Autodesk Fusion 360 part; units mm, degrees
(part 6 of 8)
  line L844 (-117.8501, 180.3501, -3) -> (-114.8501, 180.3501, -3)
  line L845 (-114.8501, 180.3501, -3) -> (-114.8501, 177.3501, -3)
  line L846 (-114.8501, 177.3501, -3) -> (-111.8501, 177.3501, -3)
  line L847 (-111.8501, 177.3501, -3) -> (-111.8501, 180.3501, -3)
  line L848 (-111.8501, 180.3501, -3) -> (-108.8501, 180.3501, -3)
  line L849 (-108.8501, 180.3501, -3) -> (-108.8501, 177.3501, -3)
  line L850 (-108.8501, 177.3501, -3) -> (-105.8501, 177.3501, -3)
  line L851 (-105.8501, 177.3501, -3) -> (-105.8501, 180.3501, -3)
  line L852 (-105.8501, 180.3501, -3) -> (-102.8501, 180.3501, -3)
  line L853 (-102.8501, 180.3501, -3) -> (-102.8501, 177.3501, -3)
  line L854 (-102.8501, 177.3501, -3) -> (-99.8501, 177.3501, -3)
  line L855 (-99.8501, 177.3501, -3) -> (-99.8501, 180.3501, -3)
  line L856 (-99.8501, 180.3501, -3) -> (-96.8501, 180.3501, -3)
  line L857 (-96.8501, 180.3501, -3) -> (-96.8501, 177.3501, -3)
  line L858 (-96.8501, 177.3501, -3) -> (-93.8501, 177.3501, -3)
  line L859 (-93.8501, 177.3501, -3) -> (-93.8501, 180.3501, -3)
  line L860 (-93.8501, 180.3501, -3) -> (-90.8501, 180.3501, -3)
  line L861 (-90.8501, 180.3501, -3) -> (-90.8501, 177.3501, -3)
  line L862 (-90.8501, 177.3501, -3) -> (-87.8501, 177.3501, -3)
  line L863 (-87.8501, 177.3501, -3) -> (-87.8501, 180.3501, -3)
  line L864 (-87.8501, 180.3501, -3) -> (-84.8501, 180.3501, -3)
  line L865 (-84.8501, 180.3501, -3) -> (-84.8501, 177.3501, -3)
  line L866 (-84.8501, 177.3501, -3) -> (-81.8501, 177.3501, -3)
  line L867 (-81.8501, 177.3501, -3) -> (-81.8501, 180.3501, -3)
  line L868 (-81.8501, 180.3501, -3) -> (-78.8501, 180.3501, -3)
  line L869 (-78.8501, 180.3501, -3) -> (-78.8501, 177.3501, -3)
  line L870 (-78.8501, 177.3501, -3) -> (-75.8501, 177.3501, -3)
  line L871 (-75.8501, 177.3501, -3) -> (-75.8501, 180.3501, -3)
  line L872 (-75.8501, 180.3501, -3) -> (-72.8501, 180.3501, -3)
  line L873 (-72.8501, 180.3501, -3) -> (-72.8501, 177.3501, -3)
  line L874 (-72.8501, 177.3501, -3) -> (-69.8501, 177.3501, -3)
  line L875 (-69.8501, 177.3501, -3) -> (-69.8501, 180.3501, -3)
  line L876 (-69.8501, 180.3501, -3) -> (-66.8501, 180.3501, -3)
  line L877 (-66.8501, 180.3501, -3) -> (-66.8501, 177.3501, -3)
  line L878 (-66.8501, 177.3501, -3) -> (-63.8501, 177.3501, -3)
  line L879 (-63.8501, 177.3501, -3) -> (-63.8501, 180.3501, -3)
  line L880 (-63.8501, 180.3501, -3) -> (-60.8501, 180.3501, -3)
  line L881 (-60.8501, 180.3501, -3) -> (-60.8501, 177.3501, -3)
  line L882 (-60.8501, 177.3501, -3) -> (-57.85, 177.3501, -3)
  line L883 (-57.85, 177.3501, -3) -> (-57.85, 180.3501, -3)
  line L884 (-57.85, 180.3501, -3) -> (-54.85, 180.3501, -3)
  line L885 (-54.85, 180.3501, -3) -> (-54.85, 177.3501, -3)
  line L886 (-54.85, 177.3501, -3) -> (-51.85, 177.3501, -3)
  line L887 (-51.85, 177.3501, -3) -> (-51.85, 180.3501, -3)
  line L888 (-51.85, 180.3501, -3) -> (-48.85, 180.3501, -3)
  line L889 (-48.85, 180.3501, -3) -> (-48.85, 177.3501, -3)
  line L890 (-48.85, 177.3501, -3) -> (-45.85, 177.3501, -3)
  line L891 (-45.85, 177.3501, -3) -> (-45.85, 180.3501, -3)
  line L892 (-45.85, 180.3501, -3) -> (-42.85, 180.3501, -3)
  line L893 (-42.85, 180.3501, -3) -> (-42.85, 177.3501, -3)
  line L894 (-42.85, 177.3501, -3) -> (-39.85, 177.3501, -3)
  line L895 (-39.85, 177.3501, -3) -> (-39.85, 180.3501, -3)
  line L896 (-39.85, 180.3501, -3) -> (-36.85, 180.3501, -3)
  line L897 (-36.85, 180.3501, -3) -> (-36.85, 177.3501, -3)
  line L898 (-36.85, 177.3501, -3) -> (-33.85, 177.3501, -3)
  line L899 (-33.85, 177.3501, -3) -> (-33.85, 180.3501, -3)
  line L900 (-33.85, 180.3501, -3) -> (-30.85, 180.3501, -3)
  line L901 (-30.85, 180.3501, -3) -> (-30.85, 177.3501, -3)
  line L902 (-30.85, 177.3501, -3) -> (-27.85, 177.3501, -3)
  line L903 (-27.85, 177.3501, -3) -> (-27.85, 180.3501, -3)
  line L904 (-27.85, 180.3501, -3) -> (-24.85, 180.3501, -3)
  line L905 (-24.85, 180.3501, -3) -> (-24.85, 177.3501, -3)
  line L906 (-24.85, 177.3501, -3) -> (-21.85, 177.3501, -3)
  line L907 (-21.85, 177.3501, -3) -> (-21.85, 180.3501, -3)
  line L908 (-21.85, 180.3501, -3) -> (-18.85, 180.3501, -3)
  line L909 (-18.85, 180.3501, -3) -> (-18.85, 177.3501, -3)
  line L910 (-18.85, 177.3501, -3) -> (-15.85, 177.3501, -3)
  line L911 (-15.85, 177.3501, -3) -> (-15.85, 180.3501, -3)
  line L912 (-15.85, 180.3501, -3) -> (-11.1, 180.3501, -3)
  line L913 (-11.1, 180.3501, -3) -> (-11.1, 177.3501, -3)
  line L914 (-11.1, 177.3501, -3) -> (-9.35, 177.3501, -3)
  line L915 (-9.35, 177.3501, -3) -> (-9.35, 176.6001, -3)
  line L916 (-9.35, 176.6001, -3) -> (-6.35, 176.6001, -3)
  line L917 (-6.35, 176.6001, -3) -> (-6.35, 172.8501, -3)
  line L918 (-6.35, 172.8501, -3) -> (-9.35, 172.8501, -3)
  line L919 (-9.35, 172.8501, -3) -> (-9.35, 169.8501, -3)
  line L920 (-9.35, 169.8501, -3) -> (-6.35, 169.8501, -3)
  line L921 (-6.35, 169.8501, -3) -> (-6.35, 166.8501, -3)
  line L922 (-6.35, 166.8501, -3) -> (-9.35, 166.8501, -3)
  line L923 (-9.35, 166.8501, -3) -> (-9.35, 163.8501, -3)
  line L924 (-9.35, 163.8501, -3) -> (-6.35, 163.8501, -3)
  line L925 (-6.35, 163.8501, -3) -> (-6.35, 160.8501, -3)
  line L926 (-6.35, 160.8501, -3) -> (-9.35, 160.8501, -3)
  line L927 (-9.35, 160.8501, -3) -> (-9.35, 157.8501, -3)
  line L928 (-9.35, 157.8501, -3) -> (-6.35, 157.8501, -3)
  line L929 (-6.35, 157.8501, -3) -> (-6.35, 154.8501, -3)
  line L930 (-6.35, 154.8501, -3) -> (-9.35, 154.8501, -3)
  line L931 (-9.35, 154.8501, -3) -> (-9.35, 151.8501, -3)
  line L932 (-9.35, 151.8501, -3) -> (-6.35, 151.8501, -3)
  line L933 (-6.35, 151.8501, -3) -> (-6.35, 148.8501, -3)
  line L934 (-6.35, 148.8501, -3) -> (-9.35, 148.8501, -3)
  line L935 (-9.35, 148.8501, -3) -> (-9.35, 145.8501, -3)
  line L936 (-9.35, 145.8501, -3) -> (-6.35, 145.8501, -3)
  line L937 (-6.35, 145.8501, -3) -> (-6.35, 142.8501, -3)
  line L938 (-6.35, 142.8501, -3) -> (-9.35, 142.8501, -3)
  line L939 (-9.35, 142.8501, -3) -> (-9.35, 139.8501, -3)
  line L940 (-9.35, 139.8501, -3) -> (-6.35, 139.8501, -3)
  line L941 (-6.35, 139.8501, -3) -> (-6.35, 136.8501, -3)
  line L942 (-6.35, 136.8501, -3) -> (-9.35, 136.8501, -3)
  line L943 (-9.35, 136.8501, -3) -> (-9.35, 133.8501, -3)
  line L944 (-9.35, 133.8501, -3) -> (-6.35, 133.8501, -3)
  line L945 (-6.35, 133.8501, -3) -> (-6.35, 130.8501, -3)
  line L946 (-6.35, 130.8501, -3) -> (-9.35, 130.8501, -3)
  line L947 (-9.35, 130.8501, -3) -> (-9.35, 127.8501, -3)
  line L948 (-9.35, 127.8501, -3) -> (-6.35, 127.8501, -3)
  line L949 (-6.35, 127.8501, -3) -> (-6.35, 124.8501, -3)
  line L950 (-6.35, 124.8501, -3) -> (-9.35, 124.8501, -3)
  line L951 (-9.35, 124.8501, -3) -> (-9.35, 121.8501, -3)
  line L952 (-9.35, 121.8501, -3) -> (-6.35, 121.8501, -3)
  line L953 (-6.35, 121.8501, -3) -> (-6.35, 118.8501, -3)
  line L954 (-6.35, 118.8501, -3) -> (-9.35, 118.8501, -3)
  line L955 (-9.35, 118.8501, -3) -> (-9.35, 115.8501, -3)
  line L956 (-9.35, 115.8501, -3) -> (-6.35, 115.8501, -3)
  line L957 (-6.35, 115.8501, -3) -> (-6.35, 112.8501, -3)
  line L958 (-6.35, 112.8501, -3) -> (-9.35, 112.8501, -3)
  line L959 (-9.35, 112.8501, -3) -> (-9.35, 109.8501, -3)
  line L960 (-9.35, 109.8501, -3) -> (-6.35, 109.8501, -3)
  line L961 (-6.35, 109.8501, -3) -> (-6.35, 106.8501, -3)
  line L962 (-6.35, 106.8501, -3) -> (-9.35, 106.8501, -3)
  line L963 (-9.35, 106.8501, -3) -> (-9.35, 103.8501, -3)
  line L964 (-9.35, 103.8501, -3) -> (-6.35, 103.8501, -3)
  line L965 (-6.35, 103.8501, -3) -> (-6.35, 100.8501, -3)
  line L966 (-6.35, 100.8501, -3) -> (-9.35, 100.8501, -3)
  line L967 (-9.35, 100.8501, -3) -> (-9.35, 97.8501, -3)
  line L968 (-9.35, 97.8501, -3) -> (-6.35, 97.8501, -3)
  line L969 (-6.35, 97.8501, -3) -> (-6.35, 94.8501, -3)
  line L970 (-6.35, 94.8501, -3) -> (-9.35, 94.8501, -3)
  line L971 (-9.35, 94.8501, -3) -> (-9.35, 91.8501, -3)
  line L972 (-9.35, 91.8501, -3) -> (-6.35, 91.8501, -3)
  line L973 (-6.35, 91.8501, -3) -> (-6.35, 88.8501, -3)
  line L974 (-6.35, 88.8501, -3) -> (-9.35, 88.8501, -3)
  line L975 (-9.35, 88.8501, -3) -> (-9.35, 85.8501, -3)
  line L976 (-9.35, 85.8501, -3) -> (-6.35, 85.8501, -3)
  line L977 (-6.35, 85.8501, -3) -> (-6.35, 82.8501, -3)
  line L978 (-6.35, 82.8501, -3) -> (-9.35, 82.8501, -3)
  line L979 (-9.35, 82.8501, -3) -> (-9.35, 79.8501, -3)
  line L980 (-9.35, 79.8501, -3) -> (-6.35, 79.8501, -3)
  line L981 (-6.35, 79.8501, -3) -> (-6.35, 76.8501, -3)
  line L982 (-6.35, 76.8501, -3) -> (-9.35, 76.8501, -3)
  line L983 (-9.35, 76.8501, -3) -> (-9.35, 73.8501, -3)
  line L984 (-9.35, 73.8501, -3) -> (-6.35, 73.8501, -3)
  line L985 (-6.35, 73.8501, -3) -> (-6.35, 70.8501, -3)
  line L986 (-6.35, 70.8501, -3) -> (-9.35, 70.8501, -3)
  line L987 (-9.35, 70.8501, -3) -> (-9.35, 67.8501, -3)
  line L988 (-9.35, 67.8501, -3) -> (-6.35, 67.8501, -3)
  line L989 (-6.35, 67.8501, -3) -> (-6.35, 64.8501, -3)
  line L990 (-6.35, 64.8501, -3) -> (-9.35, 64.8501, -3)
  line L991 (-9.35, 64.8501, -3) -> (-9.35, 61.8501, -3)
  line L992 (-9.35, 61.8501, -3) -> (-6.35, 61.8501, -3)
  line L993 (-6.35, 61.8501, -3) -> (-6.35, 58.85, -3)
  line L994 (-6.35, 58.85, -3) -> (-9.35, 58.85, -3)
  line L995 (-9.35, 58.85, -3) -> (-9.35, 55.85, -3)
  line L996 (-9.35, 55.85, -3) -> (-6.35, 55.85, -3)
  line L997 (-6.35, 55.85, -3) -> (-6.35, 52.85, -3)
  line L998 (-6.35, 52.85, -3) -> (-9.35, 52.85, -3)
  line L999 (-9.35, 52.85, -3) -> (-9.35, 49.85, -3)
  line L1000 (-9.35, 49.85, -3) -> (-6.35, 49.85, -3)
  line L1001 (-6.35, 49.85, -3) -> (-6.35, 46.85, -3)
  line L1002 (-6.35, 46.85, -3) -> (-9.35, 46.85, -3)
  line L1003 (-9.35, 46.85, -3) -> (-9.35, 43.85, -3)
  line L1004 (-9.35, 43.85, -3) -> (-6.35, 43.85, -3)
  line L1005 (-6.35, 43.85, -3) -> (-6.35, 40.85, -3)
  line L1006 (-6.35, 40.85, -3) -> (-9.35, 40.85, -3)
  line L1007 (-9.35, 40.85, -3) -> (-9.35, 37.85, -3)
  line L1008 (-9.35, 37.85, -3) -> (-6.35, 37.85, -3)
  line L1009 (-6.35, 37.85, -3) -> (-6.35, 34.85, -3)
  line L1010 (-6.35, 34.85, -3) -> (-9.35, 34.85, -3)
  line L1011 (-9.35, 34.85, -3) -> (-9.35, 31.85, -3)
  line L1012 (-9.35, 31.85, -3) -> (-6.35, 31.85, -3)
  line L1013 (-6.35, 31.85, -3) -> (-6.35, 28.1, -3)
  line L1014 (-6.35, 28.1, -3) -> (-9.35, 28.1, -3)
  line L1015 (-9.35, 28.1, -3) -> (-9.35, 27.35, -3)
  line L1016 (-9.35, 27.35, -3) -> (-11.1, 27.35, -3)
  line L1017 (-11.1, 27.35, -3) -> (-11.1, 24.35, -3)
  line L1018 (-11.1, 24.35, -3) -> (-15.85, 24.35, -3)
  line L1019 (-15.85, 24.35, -3) -> (-15.85, 27.35, -3)
  line L1020 (-15.85, 27.35, -3) -> (-18.85, 27.35, -3)
  line L1021 (-18.85, 27.35, -3) -> (-18.85, 24.35, -3)
  line L1022 (-18.85, 24.35, -3) -> (-21.85, 24.35, -3)
  line L1023 (-21.85, 24.35, -3) -> (-21.85, 27.35, -3)
  line L1024 (-21.85, 27.35, -3) -> (-24.85, 27.35, -3)
  line L1025 (-24.85, 27.35, -3) -> (-24.85, 24.35, -3)
  line L1026 (-24.85, 24.35, -3) -> (-27.85, 24.35, -3)
  line L1027 (-27.85, 24.35, -3) -> (-27.85, 27.35, -3)
  line L1028 (-27.85, 27.35, -3) -> (-30.85, 27.35, -3)
  line L1029 (-30.85, 27.35, -3) -> (-30.85, 24.35, -3)
  line L1030 (-30.85, 24.35, -3) -> (-33.85, 24.35, -3)
  line L1031 (-33.85, 24.35, -3) -> (-33.85, 27.35, -3)
  line L1032 (-33.85, 27.35, -3) -> (-36.85, 27.35, -3)
  line L1033 (-36.85, 27.35, -3) -> (-36.85, 24.35, -3)
  line L1034 (-36.85, 24.35, -3) -> (-39.85, 24.35, -3)
  line L1035 (-39.85, 24.35, -3) -> (-39.85, 27.35, -3)
  line L1036 (-39.85, 27.35, -3) -> (-42.85, 27.35, -3)
  line L1037 (-42.85, 27.35, -3) -> (-42.85, 24.35, -3)
  line L1038 (-42.85, 24.35, -3) -> (-45.85, 24.35, -3)
  line L1039 (-45.85, 24.35, -3) -> (-45.85, 27.35, -3)
  line L1040 (-45.85, 27.35, -3) -> (-48.85, 27.35, -3)
  line L1041 (-48.85, 27.35, -3) -> (-48.85, 24.35, -3)
  line L1042 (-48.85, 24.35, -3) -> (-51.85, 24.35, -3)
  line L1043 (-51.85, 24.35, -3) -> (-51.85, 27.35, -3)
  line L1044 (-51.85, 27.35, -3) -> (-54.85, 27.35, -3)
  line L1045 (-54.85, 27.35, -3) -> (-54.85, 24.35, -3)
  line L1046 (-54.85, 24.35, -3) -> (-57.85, 24.35, -3)
  line L1047 (-57.85, 24.35, -3) -> (-57.85, 27.35, -3)
  line L1048 (-57.85, 27.35, -3) -> (-60.8501, 27.35, -3)
  line L1049 (-60.8501, 27.35, -3) -> (-60.8501, 24.35, -3)
  line L1050 (-60.8501, 24.35, -3) -> (-63.8501, 24.35, -3)
  line L1051 (-63.8501, 24.35, -3) -> (-63.8501, 27.35, -3)
  line L1052 (-63.8501, 27.35, -3) -> (-66.8501, 27.35, -3)
  line L1053 (-66.8501, 27.35, -3) -> (-66.8501, 24.35, -3)
  line L1054 (-66.8501, 24.35, -3) -> (-69.8501, 24.35, -3)
  line L1055 (-69.8501, 24.35, -3) -> (-69.8501, 27.35, -3)
  line L1056 (-69.8501, 27.35, -3) -> (-72.8501, 27.35, -3)
  line L1057 (-72.8501, 27.35, -3) -> (-72.8501, 24.35, -3)
  line L1058 (-72.8501, 24.35, -3) -> (-75.8501, 24.35, -3)
  line L1059 (-75.8501, 24.35, -3) -> (-75.8501, 27.35, -3)
  line L1060 (-75.8501, 27.35, -3) -> (-78.8501, 27.35, -3)
  line L1061 (-78.8501, 27.35, -3) -> (-78.8501, 24.35, -3)
  line L1062 (-78.8501, 24.35, -3) -> (-81.8501, 24.35, -3)
  line L1063 (-81.8501, 24.35, -3) -> (-81.8501, 27.35, -3)
  line L1064 (-81.8501, 27.35, -3) -> (-84.8501, 27.35, -3)
  line L1065 (-84.8501, 27.35, -3) -> (-84.8501, 24.35, -3)
  line L1066 (-84.8501, 24.35, -3) -> (-87.8501, 24.35, -3)
  line L1067 (-87.8501, 24.35, -3) -> (-87.8501, 27.35, -3)
  line L1068 (-87.8501, 27.35, -3) -> (-90.8501, 27.35, -3)
  line L1069 (-90.8501, 27.35, -3) -> (-90.8501, 24.35, -3)
  line L1070 (-90.8501, 24.35, -3) -> (-93.8501, 24.35, -3)
  line L1071 (-93.8501, 24.35, -3) -> (-93.8501, 27.35, -3)
  line L1072 (-93.8501, 27.35, -3) -> (-96.8501, 27.35, -3)
  line L1073 (-96.8501, 27.35, -3) -> (-96.8501, 24.35, -3)
  line L1074 (-96.8501, 24.35, -3) -> (-99.8501, 24.35, -3)
  line L1075 (-99.8501, 24.35, -3) -> (-99.8501, 27.35, -3)
  line L1076 (-99.8501, 27.35, -3) -> (-102.8501, 27.35, -3)
  line L1077 (-102.8501, 27.35, -3) -> (-102.8501, 24.35, -3)
  line L1078 (-102.8501, 24.35, -3) -> (-105.8501, 24.35, -3)
  line L1079 (-105.8501, 24.35, -3) -> (-105.8501, 27.35, -3)
  line L1080 (-105.8501, 27.35, -3) -> (-108.8501, 27.35, -3)
  line L1081 (-108.8501, 27.35, -3) -> (-108.8501, 24.35, -3)
  line L1082 (-108.8501, 24.35, -3) -> (-111.8501, 24.35, -3)
  line L1083 (-111.8501, 24.35, -3) -> (-111.8501, 27.35, -3)
  line L1084 (-111.8501, 27.35, -3) -> (-114.8501, 27.35, -3)
  line L1085 (-114.8501, 27.35, -3) -> (-114.8501, 24.35, -3)
  line L1086 (-114.8501, 24.35, -3) -> (-117.8501, 24.35, -3)
  line L1087 (-117.8501, 24.35, -3) -> (-117.8501, 27.35, -3)
  line L1088 (-117.8501, 27.35, -3) -> (-120.8501, 27.35, -3)
  line L1089 (-120.8501, 27.35, -3) -> (-120.8501, 24.35, -3)
  line L1090 (-120.8501, 24.35, -3) -> (-123.8501, 24.35, -3)
  line L1091 (-123.8501, 24.35, -3) -> (-123.8501, 27.35, -3)
  line L1092 (-123.8501, 27.35, -3) -> (-126.8501, 27.35, -3)
  line L1093 (-126.8501, 27.35, -3) -> (-126.8501, 24.35, -3)
  line L1094 (-126.8501, 24.35, -3) -> (-129.8501, 24.35, -3)
  line L1095 (-129.8501, 24.35, -3) -> (-129.8501, 27.35, -3)
  line L1096 (-129.8501, 27.35, -3) -> (-132.8501, 27.35, -3)
  line L1097 (-132.8501, 27.35, -3) -> (-132.8501, 24.35, -3)
  line L1098 (-132.8501, 24.35, -3) -> (-135.8501, 24.35, -3)
  line L1099 (-135.8501, 24.35, -3) -> (-135.8501, 27.35, -3)
  line L1100 (-135.8501, 27.35, -3) -> (-138.8501, 27.35, -3)
  line L1101 (-138.8501, 27.35, -3) -> (-138.8501, 24.35, -3)
  line L1102 (-138.8501, 24.35, -3) -> (-141.8501, 24.35, -3)
  line L1103 (-141.8501, 24.35, -3) -> (-141.8501, 27.35, -3)
  line L1104 (-141.8501, 27.35, -3) -> (-144.8501, 27.35, -3)
  line L1105 (-144.8501, 27.35, -3) -> (-144.8501, 24.35, -3)
  line L1106 (-144.8501, 24.35, -3) -> (-147.8501, 24.35, -3)
  line L1107 (-147.8501, 24.35, -3) -> (-147.8501, 27.35, -3)
  line L1108 (-147.8501, 27.35, -3) -> (-150.8501, 27.35, -3)
  line L1109 (-150.8501, 27.35, -3) -> (-150.8501, 24.35, -3)
  line L1110 (-150.8501, 24.35, -3) -> (-153.8501, 24.35, -3)
  line L1111 (-153.8501, 24.35, -3) -> (-153.8501, 27.35, -3)
  line L1112 (-153.8501, 27.35, -3) -> (-156.8501, 27.35, -3)
  line L1113 (-156.8501, 27.35, -3) -> (-156.8501, 24.35, -3)
  line L1114 (-156.8501, 24.35, -3) -> (-159.8501, 24.35, -3)
  line L1115 (-159.8501, 24.35, -3) -> (-159.8501, 27.35, -3)
  line L1116 (-159.8501, 27.35, -3) -> (-162.8501, 27.35, -3)
  line L1117 (-162.8501, 27.35, -3) -> (-162.8501, 24.35, -3)
  line L1118 (-162.8501, 24.35, -3) -> (-165.8501, 24.35, -3)
  line L1119 (-165.8501, 24.35, -3) -> (-165.8501, 27.35, -3)
  line L1120 (-165.8501, 27.35, -3) -> (-168.8501, 27.35, -3)
  line L1121 (-168.8501, 27.35, -3) -> (-168.8501, 24.35, -3)
  line L1122 (-168.8501, 24.35, -3) -> (-171.8501, 24.35, -3)
  line L1123 (-171.8501, 24.35, -3) -> (-171.8501, 27.35, -3)
  line L1124 (-171.8501, 27.35, -3) -> (-174.8501, 27.35, -3)
  line L1125 (-174.8501, 27.35, -3) -> (-174.8501, 24.35, -3)
  line L1126 (-174.8501, 24.35, -3) -> (-177.8501, 24.35, -3)
  line L1127 (-177.8501, 24.35, -3) -> (-177.8501, 27.35, -3)
  line L1128 (-177.8501, 27.35, -3) -> (-180.8501, 27.35, -3)
  line L1129 (-180.8501, 27.35, -3) -> (-180.8501, 24.35, -3)
  line L1130 (-180.8501, 24.35, -3) -> (-183.8502, 24.35, -3)
  line L1131 (-183.8502, 24.35, -3) -> (-183.8502, 27.35, -3)
  line L1132 (-183.8502, 27.35, -3) -> (-186.8502, 27.35, -3)
  line L1133 (-186.8502, 27.35, -3) -> (-186.8502, 24.35, -3)
  line L1134 (-186.8502, 24.35, -3) -> (-189.8502, 24.35, -3)
  line L1135 (-189.8502, 24.35, -3) -> (-189.8502, 27.35, -3)
  line L1136 (-189.8502, 27.35, -3) -> (-192.8502, 27.35, -3)
  line L1137 (-192.8502, 27.35, -3) -> (-192.8502, 24.35, -3)
  line L1138 (-192.8502, 24.35, -3) -> (-195.8502, 24.35, -3)
  line L1139 (-195.8502, 24.35, -3) -> (-195.8502, 27.35, -3)
  line L1140 (-195.8502, 27.35, -3) -> (-198.8502, 27.35, -3)
  line L1141 (-198.8502, 27.35, -3) -> (-198.8502, 24.35, -3)
  line L1142 (-198.8502, 24.35, -3) -> (-201.8502, 24.35, -3)
  line L1143 (-201.8502, 24.35, -3) -> (-201.8502, 27.35, -3)
  line L1144 (-201.8502, 27.35, -3) -> (-204.8502, 27.35, -3)
  line L1145 (-204.8502, 27.35, -3) -> (-204.8502, 24.35, -3)
  line L1146 (-204.8502, 24.35, -3) -> (-207.8502, 24.35, -3)
  line L1147 (-207.8502, 24.35, -3) -> (-207.8502, 27.35, -3)
  line L1148 (-207.8502, 27.35, -3) -> (-210.8502, 27.35, -3)
  line L1149 (-210.8502, 27.35, -3) -> (-210.8502, 24.35, -3)
  line L1150 (-210.8502, 24.35, -3) -> (-213.8502, 24.35, -3)
  line L1151 (-213.8502, 24.35, -3) -> (-213.8502, 27.35, -3)
  line L1152 (-213.8502, 27.35, -3) -> (-216.8502, 27.35, -3)
  line L1153 (-216.8502, 27.35, -3) -> (-216.8502, 24.35, -3)
  line L1154 (-216.8502, 24.35, -3) -> (-219.8502, 24.35, -3)
  line L1155 (-219.8502, 24.35, -3) -> (-219.8502, 27.35, -3)
  line L1156 (-219.8502, 27.35, -3) -> (-222.8502, 27.35, -3)
  line L1157 (-222.8502, 27.35, -3) -> (-222.8502, 24.35, -3)
  line L1158 (-222.8502, 24.35, -3) -> (-225.8502, 24.35, -3)
  line L1159 (-225.8502, 24.35, -3) -> (-225.8502, 27.35, -3)
  line L1160 (-225.8502, 27.35, -3) -> (-228.8502, 27.35, -3)
  line L1161 (-228.8502, 27.35, -3) -> (-228.8502, 24.35, -3)
  line L1162 (-228.8502, 24.35, -3) -> (-231.8502, 24.35, -3)
  line L1163 (-231.8502, 24.35, -3) -> (-231.8502, 27.35, -3)
  line L1164 (-231.8502, 27.35, -3) -> (-234.8502, 27.35, -3)
  line L1165 (-234.8502, 27.35, -3) -> (-234.8502, 24.35, -3)
  line L1166 (-234.8502, 24.35, -3) -> (-237.8502, 24.35, -3)
  line L1167 (-237.8502, 24.35, -3) -> (-237.8502, 27.35, -3)
  line L1168 (-237.8502, 27.35, -3) -> (-240.8502, 27.35, -3)
  line L1169 (-240.8502, 27.35, -3) -> (-240.8502, 24.35, -3)
  line L1170 (-240.8502, 24.35, -3) -> (-243.8502, 24.35, -3)
  line L1171 (-243.8502, 24.35, -3) -> (-243.8502, 27.35, -3)
  line L1172 (-243.8502, 27.35, -3) -> (-246.8502, 27.35, -3)
  line L1173 (-246.8502, 27.35, -3) -> (-246.8502, 24.35, -3)
  line L1174 (-246.8502, 24.35, -3) -> (-249.8502, 24.35, -3)
  line L1175 (-249.8502, 24.35, -3) -> (-249.8502, 27.35, -3)
  line L1176 (-249.8502, 27.35, -3) -> (-252.8502, 27.35, -3)
  line L1177 (-252.8502, 27.35, -3) -> (-252.8502, 24.35, -3)
  line L1178 (-252.8502, 24.35, -3) -> (-255.8502, 24.35, -3)
  line L1179 (-255.8502, 24.35, -3) -> (-255.8502, 27.35, -3)
  line L1180 (-255.8502, 27.35, -3) -> (-258.8502, 27.35, -3)
  line L1181 (-258.8502, 27.35, -3) -> (-258.8502, 24.35, -3)
  line L1182 (-258.8502, 24.35, -3) -> (-261.8502, 24.35, -3)
  line L1183 (-261.8502, 24.35, -3) -> (-261.8502, 27.35, -3)
  line L1184 (-261.8502, 27.35, -3) -> (-264.8502, 27.35, -3)
  line L1185 (-264.8502, 27.35, -3) -> (-264.8502, 24.35, -3)
  line L1186 (-264.8502, 24.35, -3) -> (-267.8502, 24.35, -3)
  line L1187 (-267.8502, 24.35, -3) -> (-267.8502, 27.35, -3)
  line L1188 (-267.8502, 27.35, -3) -> (-270.8502, 27.35, -3)
  line L1189 (-270.8502, 27.35, -3) -> (-270.8502, 24.35, -3)
  line L1190 (-270.8502, 24.35, -3) -> (-273.8502, 24.35, -3)
  line L1191 (-273.8502, 24.35, -3) -> (-273.8502, 27.35, -3)
  line L1192 (-273.8502, 27.35, -3) -> (-276.8502, 27.35, -3)
  line L1193 (-276.8502, 27.35, -3) -> (-276.8502, 24.35, -3)
  line L1194 (-276.8502, 24.35, -3) -> (-279.8502, 24.35, -3)
  line L1195 (-279.8502, 24.35, -3) -> (-279.8502, 27.35, -3)
  line L1196 (-279.8502, 27.35, -3) -> (-282.8502, 27.35, -3)
  line L1197 (-282.8502, 27.35, -3) -> (-282.8502, 24.35, -3)
  line L1198 (-282.8502, 24.35, -3) -> (-285.8502, 24.35, -3)
  line L1199 (-285.8502, 24.35, -3) -> (-285.8502, 27.35, -3)
  line L1200 (-285.8502, 27.35, -3) -> (-288.8502, 27.35, -3)
  line L1201 (-288.8502, 27.35, -3) -> (-288.8502, 24.35, -3)
  line L1202 (-288.8502, 24.35, -3) -> (-291.8502, 24.35, -3)
  line L1203 (-291.8502, 24.35, -3) -> (-291.8502, 27.35, -3)
  line L1204 (-291.8502, 27.35, -3) -> (-294.8502, 27.35, -3)
  line L1205 (-294.8502, 27.35, -3) -> (-294.8502, 24.35, -3)
  line L1206 (-294.8502, 24.35, -3) -> (-297.8502, 24.35, -3)
  line L1207 (-297.8502, 24.35, -3) -> (-297.8502, 27.35, -3)
  line L1208 (-297.8502, 27.35, -3) -> (-300.8502, 27.35, -3)
  line L1209 (-300.8502, 27.35, -3) -> (-300.8502, 24.35, -3)
  line L1210 (-300.8502, 24.35, -3) -> (-303.8502, 24.35, -3)
  line L1211 (-303.8502, 24.35, -3) -> (-303.8502, 27.35, -3)
  line L1212 (-303.8502, 27.35, -3) -> (-306.8503, 27.35, -3)
  line L1213 (-306.8503, 27.35, -3) -> (-306.8503, 24.35, -3)
  line L1214 (-306.8503, 24.35, -3) -> (-309.8503, 24.35, -3)
  line L1215 (-309.8503, 24.35, -3) -> (-309.8503, 27.35, -3)
  line L1216 (-309.8503, 27.35, -3) -> (-312.8503, 27.35, -3)
  line L1217 (-312.8503, 27.35, -3) -> (-312.8503, 24.35, -3)
  line L1218 (-312.8503, 24.35, -3) -> (-317.6003, 24.35, -3)
  line L1219 (-317.6003, 24.35, -3) -> (-317.6003, 27.35, -3)
  line L1220 (-317.6003, 27.35, -3) -> (-319.3503, 27.35, -3)
  line L1221 (-319.3503, 27.35, -3) -> (-319.3503, 28.1, -3)
  line L1222 (-319.3503, 28.1, -3) -> (-322.3503, 28.1, -3)
  line L1223 (-322.3503, 28.1, -3) -> (-322.3503, 31.85, -3)
  line L1224 (-319.3503, 10.1) -> (-322.3503, 10.1)
  line L1225 (-322.3503, 10.1) -> (-322.3503, 6.35)
  line L1226 (-322.3503, 6.35) -> (-317.6003, 6.35)
  line L1227 (-317.6003, 6.35) -> (-317.6003, 9.35)
  line L1228 (-317.6003, 9.35) -> (-312.8503, 9.35)
  line L1229 (-312.8503, 9.35) -> (-312.8503, 6.35)
  line L1230 (-312.8503, 6.35) -> (-309.8503, 6.35)
  line L1231 (-309.8503, 6.35) -> (-309.8503, 9.35)
  line L1232 (-309.8503, 9.35) -> (-306.8503, 9.35)
  line L1233 (-306.8503, 9.35) -> (-306.8503, 6.35)
  line L1234 (-306.8503, 6.35) -> (-303.8502, 6.35)
  line L1235 (-303.8502, 6.35) -> (-303.8502, 9.35)
  line L1236 (-303.8502, 9.35) -> (-300.8502, 9.35)
  line L1237 (-300.8502, 9.35) -> (-300.8502, 6.35)
  line L1238 (-300.8502, 6.35) -> (-297.8502, 6.35)
  line L1239 (-297.8502, 6.35) -> (-297.8502, 9.35)
  line L1240 (-297.8502, 9.35) -> (-294.8502, 9.35)
  line L1241 (-294.8502, 9.35) -> (-294.8502, 6.35)
  line L1242 (-294.8502, 6.35) -> (-291.8502, 6.35)
  line L1243 (-291.8502, 6.35) -> (-291.8502, 9.35)
  line L1244 (-291.8502, 9.35) -> (-288.8502, 9.35)
  line L1245 (-288.8502, 9.35) -> (-288.8502, 6.35)
  line L1246 (-288.8502, 6.35) -> (-285.8502, 6.35)
  line L1247 (-285.8502, 6.35) -> (-285.8502, 9.35)
  line L1248 (-285.8502, 9.35) -> (-282.8502, 9.35)
  line L1249 (-282.8502, 9.35) -> (-282.8502, 6.35)
  line L1250 (-282.8502, 6.35) -> (-279.8502, 6.35)
  line L1251 (-279.8502, 6.35) -> (-279.8502, 9.35)
  line L1252 (-279.8502, 9.35) -> (-276.8502, 9.35)
  line L1253 (-276.8502, 9.35) -> (-276.8502, 6.35)
  line L1254 (-276.8502, 6.35) -> (-273.8502, 6.35)
  line L1255 (-273.8502, 6.35) -> (-273.8502, 9.35)
  line L1256 (-273.8502, 9.35) -> (-270.8502, 9.35)
  line L1257 (-270.8502, 9.35) -> (-270.8502, 6.35)
  line L1258 (-270.8502, 6.35) -> (-267.8502, 6.35)
  line L1259 (-267.8502, 6.35) -> (-267.8502, 9.35)
  line L1260 (-267.8502, 9.35) -> (-264.8502, 9.35)
  line L1261 (-264.8502, 9.35) -> (-264.8502, 6.35)
  line L1262 (-264.8502, 6.35) -> (-261.8502, 6.35)
  line L1263 (-261.8502, 6.35) -> (-261.8502, 9.35)
  line L1264 (-261.8502, 9.35) -> (-258.8502, 9.35)
  line L1265 (-258.8502, 9.35) -> (-258.8502, 6.35)
  line L1266 (-258.8502, 6.35) -> (-255.8502, 6.35)
  line L1267 (-255.8502, 6.35) -> (-255.8502, 9.35)
  line L1268 (-255.8502, 9.35) -> (-252.8502, 9.35)
  line L1269 (-252.8502, 9.35) -> (-252.8502, 6.35)
  line L1270 (-252.8502, 6.35) -> (-249.8502, 6.35)
  line L1271 (-249.8502, 6.35) -> (-249.8502, 9.35)
  line L1272 (-249.8502, 9.35) -> (-246.8502, 9.35)
  line L1273 (-246.8502, 9.35) -> (-246.8502, 6.35)
  line L1274 (-246.8502, 6.35) -> (-243.8502, 6.35)
  line L1275 (-243.8502, 6.35) -> (-243.8502, 9.35)
  line L1276 (-243.8502, 9.35) -> (-240.8502, 9.35)
  line L1277 (-240.8502, 9.35) -> (-240.8502, 6.35)
  line L1278 (-240.8502, 6.35) -> (-237.8502, 6.35)
  line L1279 (-237.8502, 6.35) -> (-237.8502, 9.35)
  line L1280 (-237.8502, 9.35) -> (-234.8502, 9.35)
  line L1281 (-234.8502, 9.35) -> (-234.8502, 6.35)
  line L1282 (-234.8502, 6.35) -> (-231.8502, 6.35)
  line L1283 (-231.8502, 6.35) -> (-231.8502, 9.35)
  line L1284 (-231.8502, 9.35) -> (-228.8502, 9.35)
  line L1285 (-228.8502, 9.35) -> (-228.8502, 6.35)
  line L1286 (-228.8502, 6.35) -> (-225.8502, 6.35)
  line L1287 (-225.8502, 6.35) -> (-225.8502, 9.35)
  line L1288 (-225.8502, 9.35) -> (-222.8502, 9.35)
  line L1289 (-222.8502, 9.35) -> (-222.8502, 6.35)
  line L1290 (-222.8502, 6.35) -> (-219.8502, 6.35)
  line L1291 (-219.8502, 6.35) -> (-219.8502, 9.35)
  line L1292 (-219.8502, 9.35) -> (-216.8502, 9.35)
  line L1293 (-216.8502, 9.35) -> (-216.8502, 6.35)
  line L1294 (-216.8502, 6.35) -> (-213.8502, 6.35)
  line L1295 (-213.8502, 6.35) -> (-213.8502, 9.35)
  line L1296 (-213.8502, 9.35) -> (-210.8502, 9.35)
  line L1297 (-210.8502, 9.35) -> (-210.8502, 6.35)
  line L1298 (-210.8502, 6.35) -> (-207.8502, 6.35)
  line L1299 (-207.8502, 6.35) -> (-207.8502, 9.35)
  line L1300 (-207.8502, 9.35) -> (-204.8502, 9.35)
  line L1301 (-204.8502, 9.35) -> (-204.8502, 6.35)
  line L1302 (-204.8502, 6.35) -> (-201.8502, 6.35)
  line L1303 (-201.8502, 6.35) -> (-201.8502, 9.35)
  line L1304 (-201.8502, 9.35) -> (-198.8502, 9.35)
  line L1305 (-198.8502, 9.35) -> (-198.8502, 6.35)
  line L1306 (-198.8502, 6.35) -> (-195.8502, 6.35)
  line L1307 (-195.8502, 6.35) -> (-195.8502, 9.35)
  line L1308 (-195.8502, 9.35) -> (-192.8502, 9.35)
  line L1309 (-192.8502, 9.35) -> (-192.8502, 6.35)
  line L1310 (-192.8502, 6.35) -> (-189.8502, 6.35)
  line L1311 (-189.8502, 6.35) -> (-189.8502, 9.35)
  line L1312 (-189.8502, 9.35) -> (-186.8502, 9.35)
  line L1313 (-186.8502, 9.35) -> (-186.8502, 6.35)
  line L1314 (-186.8502, 6.35) -> (-183.8502, 6.35)
  line L1315 (-183.8502, 6.35) -> (-183.8502, 9.35)
  line L1316 (-183.8502, 9.35) -> (-180.8501, 9.35)
  line L1317 (-180.8501, 9.35) -> (-180.8501, 6.35)
  line L1318 (-180.8501, 6.35) -> (-177.8501, 6.35)
  line L1319 (-177.8501, 6.35) -> (-177.8501, 9.35)
  line L1320 (-177.8501, 9.35) -> (-174.8501, 9.35)
  line L1321 (-174.8501, 9.35) -> (-174.8501, 6.35)
  line L1322 (-174.8501, 6.35) -> (-171.8501, 6.35)
  line L1323 (-171.8501, 6.35) -> (-171.8501, 9.35)
  line L1324 (-171.8501, 9.35) -> (-168.8501, 9.35)
  line L1325 (-168.8501, 9.35) -> (-168.8501, 6.35)
  line L1326 (-168.8501, 6.35) -> (-165.8501, 6.35)
  line L1327 (-165.8501, 6.35) -> (-165.8501, 9.35)
  line L1328 (-165.8501, 9.35) -> (-162.8501, 9.35)
  line L1329 (-162.8501, 9.35) -> (-162.8501, 6.35)
  line L1330 (-162.8501, 6.35) -> (-159.8501, 6.35)
  line L1331 (-159.8501, 6.35) -> (-159.8501, 9.35)
  line L1332 (-159.8501, 9.35) -> (-156.8501, 9.35)
  line L1333 (-156.8501, 9.35) -> (-156.8501, 6.35)
  line L1334 (-156.8501, 6.35) -> (-153.8501, 6.35)
  line L1335 (-153.8501, 6.35) -> (-153.8501, 9.35)
  line L1336 (-153.8501, 9.35) -> (-150.8501, 9.35)
  line L1337 (-150.8501, 9.35) -> (-150.8501, 6.35)
  line L1338 (-150.8501, 6.35) -> (-147.8501, 6.35)
  line L1339 (-147.8501, 6.35) -> (-147.8501, 9.35)
  line L1340 (-147.8501, 9.35) -> (-144.8501, 9.35)
  line L1341 (-144.8501, 9.35) -> (-144.8501, 6.35)
  line L1342 (-144.8501, 6.35) -> (-141.8501, 6.35)
  line L1343 (-141.8501, 6.35) -> (-141.8501, 9.35)
  line L1344 (-141.8501, 9.35) -> (-138.8501, 9.35)
  line L1345 (-138.8501, 9.35) -> (-138.8501, 6.35)
  line L1346 (-138.8501, 6.35) -> (-135.8501, 6.35)
  line L1347 (-135.8501, 6.35) -> (-135.8501, 9.35)
  line L1348 (-135.8501, 9.35) -> (-132.8501, 9.35)
  line L1349 (-132.8501, 9.35) -> (-132.8501, 6.35)
  line L1350 (-132.8501, 6.35) -> (-129.8501, 6.35)
  line L1351 (-129.8501, 6.35) -> (-129.8501, 9.35)
  line L1352 (-129.8501, 9.35) -> (-126.8501, 9.35)
  line L1353 (-126.8501, 9.35) -> (-126.8501, 6.35)
  line L1354 (-126.8501, 6.35) -> (-123.8501, 6.35)
  line L1355 (-123.8501, 6.35) -> (-123.8501, 9.35)
  line L1356 (-123.8501, 9.35) -> (-120.8501, 9.35)
  line L1357 (-120.8501, 9.35) -> (-120.8501, 6.35)
  line L1358 (-120.8501, 6.35) -> (-117.8501, 6.35)
  line L1359 (-117.8501, 6.35) -> (-117.8501, 9.35)
  line L1360 (-117.8501, 9.35) -> (-114.8501, 9.35)
  line L1361 (-114.8501, 9.35) -> (-114.8501, 6.35)
  line L1362 (-114.8501, 6.35) -> (-111.8501, 6.35)
  line L1363 (-111.8501, 6.35) -> (-111.8501, 9.35)
  line L1364 (-111.8501, 9.35) -> (-108.8501, 9.35)
  line L1365 (-108.8501, 9.35) -> (-108.8501, 6.35)
  line L1366 (-108.8501, 6.35) -> (-105.8501, 6.35)
  line L1367 (-105.8501, 6.35) -> (-105.8501, 9.35)
  line L1368 (-105.8501, 9.35) -> (-102.8501, 9.35)
  line L1369 (-102.8501, 9.35) -> (-102.8501, 6.35)
  line L1370 (-102.8501, 6.35) -> (-99.8501, 6.35)
  line L1371 (-99.8501, 6.35) -> (-99.8501, 9.35)
  line L1372 (-99.8501, 9.35) -> (-96.8501, 9.35)
  line L1373 (-96.8501, 9.35) -> (-96.8501, 6.35)
  line L1374 (-96.8501, 6.35) -> (-93.8501, 6.35)
  line L1375 (-93.8501, 6.35) -> (-93.8501, 9.35)
  line L1376 (-93.8501, 9.35) -> (-90.8501, 9.35)
  line L1377 (-90.8501, 9.35) -> (-90.8501, 6.35)
  line L1378 (-90.8501, 6.35) -> (-87.8501, 6.35)
  line L1379 (-87.8501, 6.35) -> (-87.8501, 9.35)
  line L1380 (-87.8501, 9.35) -> (-84.8501, 9.35)
  line L1381 (-84.8501, 9.35) -> (-84.8501, 6.35)
  line L1382 (-84.8501, 6.35) -> (-81.8501, 6.35)
  line L1383 (-81.8501, 6.35) -> (-81.8501, 9.35)
  line L1384 (-81.8501, 9.35) -> (-78.8501, 9.35)
  line L1385 (-78.8501, 9.35) -> (-78.8501, 6.35)
  line L1386 (-78.8501, 6.35) -> (-75.8501, 6.35)
  line L1387 (-75.8501, 6.35) -> (-75.8501, 9.35)
  line L1388 (-75.8501, 9.35) -> (-72.8501, 9.35)
  line L1389 (-72.8501, 9.35) -> (-72.8501, 6.35)
  line L1390 (-72.8501, 6.35) -> (-69.8501, 6.35)
  line L1391 (-69.8501, 6.35) -> (-69.8501, 9.35)
  line L1392 (-69.8501, 9.35) -> (-66.8501, 9.35)
  line L1393 (-66.8501, 9.35) -> (-66.8501, 6.35)
  line L1394 (-66.8501, 6.35) -> (-63.8501, 6.35)
  line L1395 (-63.8501, 6.35) -> (-63.8501, 9.35)
  line L1396 (-63.8501, 9.35) -> (-60.8501, 9.35)
  line L1397 (-60.8501, 9.35) -> (-60.8501, 6.35)
  line L1398 (-60.8501, 6.35) -> (-57.85, 6.35)
  line L1399 (-57.85, 6.35) -> (-57.85, 9.35)
  line L1400 (-57.85, 9.35) -> (-54.85, 9.35)
  line L1401 (-54.85, 9.35) -> (-54.85, 6.35)
  line L1402 (-54.85, 6.35) -> (-51.85, 6.35)
  line L1403 (-51.85, 6.35) -> (-51.85, 9.35)
  line L1404 (-51.85, 9.35) -> (-48.85, 9.35)
  line L1405 (-48.85, 9.35) -> (-48.85, 6.35)
  line L1406 (-48.85, 6.35) -> (-45.85, 6.35)
  line L1407 (-45.85, 6.35) -> (-45.85, 9.35)
  line L1408 (-45.85, 9.35) -> (-42.85, 9.35)
  line L1409 (-42.85, 9.35) -> (-42.85, 6.35)
  line L1410 (-42.85, 6.35) -> (-39.85, 6.35)
  line L1411 (-39.85, 6.35) -> (-39.85, 9.35)
  line L1412 (-39.85, 9.35) -> (-36.85, 9.35)
  line L1413 (-36.85, 9.35) -> (-36.85, 6.35)
  line L1414 (-36.85, 6.35) -> (-33.85, 6.35)
  line L1415 (-33.85, 6.35) -> (-33.85, 9.35)
  line L1416 (-33.85, 9.35) -> (-30.85, 9.35)
  line L1417 (-30.85, 9.35) -> (-30.85, 6.35)
  line L1418 (-30.85, 6.35) -> (-27.85, 6.35)
  line L1419 (-27.85, 6.35) -> (-27.85, 9.35)
  line L1420 (-27.85, 9.35) -> (-24.85, 9.35)
  line L1421 (-24.85, 9.35) -> (-24.85, 6.35)
  line L1422 (-24.85, 6.35) -> (-21.85, 6.35)
  line L1423 (-21.85, 6.35) -> (-21.85, 9.35)
  line L1424 (-21.85, 9.35) -> (-18.85, 9.35)
  line L1425 (-18.85, 9.35) -> (-18.85, 6.35)
  line L1426 (-18.85, 6.35) -> (-15.85, 6.35)
  line L1427 (-15.85, 6.35) -> (-15.85, 9.35)
  line L1428 (-15.85, 9.35) -> (-11.1, 9.35)
  line L1429 (-11.1, 9.35) -> (-11.1, 6.35)
  line L1430 (-11.1, 6.35) -> (-6.35, 6.35)
  line L1431 (-6.35, 6.35) -> (-6.35, 10.1)
  line L1432 (-6.35, 10.1) -> (-9.35, 10.1)
  line L1433 (-9.35, 10.1) -> (-9.35, 13.85)
  line L1434 (-9.35, 13.85) -> (-6.35, 13.85)
  line L1435 (-6.35, 13.85) -> (-6.35, 16.85)
  line L1436 (-6.35, 16.85) -> (-9.35, 16.85)
  line L1437 (-9.35, 16.85) -> (-9.35, 20.6)
  line L1438 (-9.35, 20.6) -> (-6.35, 20.6)
  line L1439 (-6.35, 20.6) -> (-6.35, 24.35)
  line L1440 (-6.35, 24.35) -> (-11.1, 24.35)
  line L1441 (-11.1, 24.35) -> (-11.1, 21.35)
  line L1442 (-11.1, 21.35) -> (-15.85, 21.35)
  line L1443 (-15.85, 21.35) -> (-15.85, 24.35)
  line L1444 (-15.85, 24.35) -> (-18.85, 24.35)
  line L1445 (-18.85, 24.35) -> (-18.85, 21.35)
  line L1446 (-18.85, 21.35) -> (-21.85, 21.35)
  line L1447 (-21.85, 21.35) -> (-21.85, 24.35)
  line L1448 (-21.85, 24.35) -> (-24.85, 24.35)
  line L1449 (-24.85, 24.35) -> (-24.85, 21.35)
  line L1450 (-24.85, 21.35) -> (-27.85, 21.35)
  line L1451 (-27.85, 21.35) -> (-27.85, 24.35)
  line L1452 (-27.85, 24.35) -> (-30.85, 24.35)
  line L1453 (-30.85, 24.35) -> (-30.85, 21.35)
  line L1454 (-30.85, 21.35) -> (-33.85, 21.35)
  line L1455 (-33.85, 21.35) -> (-33.85, 24.35)
  line L1456 (-33.85, 24.35) -> (-36.85, 24.35)
  line L1457 (-36.85, 24.35) -> (-36.85, 21.35)
  line L1458 (-36.85, 21.35) -> (-39.85, 21.35)
  line L1459 (-39.85, 21.35) -> (-39.85, 24.35)
  line L1460 (-39.85, 24.35) -> (-42.85, 24.35)
  line L1461 (-42.85, 24.35) -> (-42.85, 21.35)
  line L1462 (-42.85, 21.35) -> (-45.85, 21.35)
  line L1463 (-45.85, 21.35) -> (-45.85, 24.35)
  line L1464 (-45.85, 24.35) -> (-48.85, 24.35)
  line L1465 (-48.85, 24.35) -> (-48.85, 21.35)
  line L1466 (-48.85, 21.35) -> (-51.85, 21.35)
  line L1467 (-51.85, 21.35) -> (-51.85, 24.35)
  line L1468 (-51.85, 24.35) -> (-54.85, 24.35)
  line L1469 (-54.85, 24.35) -> (-54.85, 21.35)
  line L1470 (-54.85, 21.35) -> (-57.85, 21.35)
  line L1471 (-57.85, 21.35) -> (-57.85, 24.35)
  line L1472 (-57.85, 24.35) -> (-60.8501, 24.35)
  line L1473 (-60.8501, 24.35) -> (-60.8501, 21.35)
  line L1474 (-60.8501, 21.35) -> (-63.8501, 21.35)
  line L1475 (-63.8501, 21.35) -> (-63.8501, 24.35)
  line L1476 (-63.8501, 24.35) -> (-66.8501, 24.35)
  line L1477 (-66.8501, 24.35) -> (-66.8501, 21.35)
  line L1478 (-66.8501, 21.35) -> (-69.8501, 21.35)
  line L1479 (-69.8501, 21.35) -> (-69.8501, 24.35)
  line L1480 (-69.8501, 24.35) -> (-72.8501, 24.35)
  line L1481 (-72.8501, 24.35) -> (-72.8501, 21.35)
  line L1482 (-72.8501, 21.35) -> (-75.8501, 21.35)
  line L1483 (-75.8501, 21.35) -> (-75.8501, 24.35)
  line L1484 (-75.8501, 24.35) -> (-78.8501, 24.35)
  line L1485 (-78.8501, 24.35) -> (-78.8501, 21.35)
  line L1486 (-78.8501, 21.35) -> (-81.8501, 21.35)
  line L1487 (-81.8501, 21.35) -> (-81.8501, 24.35)
  line L1488 (-81.8501, 24.35) -> (-84.8501, 24.35)
  line L1489 (-84.8501, 24.35) -> (-84.8501, 21.35)
  line L1490 (-84.8501, 21.35) -> (-87.8501, 21.35)
  line L1491 (-87.8501, 21.35) -> (-87.8501, 24.35)
  line L1492 (-87.8501, 24.35) -> (-90.8501, 24.35)
  line L1493 (-90.8501, 24.35) -> (-90.8501, 21.35)
  line L1494 (-90.8501, 21.35) -> (-93.8501, 21.35)
  line L1495 (-93.8501, 21.35) -> (-93.8501, 24.35)
  line L1496 (-93.8501, 24.35) -> (-96.8501, 24.35)
  line L1497 (-96.8501, 24.35) -> (-96.8501, 21.35)
  line L1498 (-96.8501, 21.35) -> (-99.8501, 21.35)
  line L1499 (-99.8501, 21.35) -> (-99.8501, 24.35)
  line L1500 (-99.8501, 24.35) -> (-102.8501, 24.35)
  line L1501 (-102.8501, 24.35) -> (-102.8501, 21.35)
  line L1502 (-102.8501, 21.35) -> (-105.8501, 21.35)
  line L1503 (-105.8501, 21.35) -> (-105.8501, 24.35)
  line L1504 (-105.8501, 24.35) -> (-108.8501, 24.35)
  line L1505 (-108.8501, 24.35) -> (-108.8501, 21.35)
  line L1506 (-108.8501, 21.35) -> (-111.8501, 21.35)
  line L1507 (-111.8501, 21.35) -> (-111.8501, 24.35)
  line L1508 (-111.8501, 24.35) -> (-114.8501, 24.35)
  line L1509 (-114.8501, 24.35) -> (-114.8501, 21.35)
  line L1510 (-114.8501, 21.35) -> (-117.8501, 21.35)
  line L1511 (-117.8501, 21.35) -> (-117.8501, 24.35)
  line L1512 (-117.8501, 24.35) -> (-120.8501, 24.35)
  line L1513 (-120.8501, 24.35) -> (-120.8501, 21.35)
  line L1514 (-120.8501, 21.35) -> (-123.8501, 21.35)
  line L1515 (-123.8501, 21.35) -> (-123.8501, 24.35)
  line L1516 (-123.8501, 24.35) -> (-126.8501, 24.35)
  line L1517 (-126.8501, 24.35) -> (-126.8501, 21.35)
  line L1518 (-126.8501, 21.35) -> (-129.8501, 21.35)
  line L1519 (-129.8501, 21.35) -> (-129.8501, 24.35)
  line L1520 (-129.8501, 24.35) -> (-132.8501, 24.35)
  line L1521 (-132.8501, 24.35) -> (-132.8501, 21.35)
  line L1522 (-132.8501, 21.35) -> (-135.8501, 21.35)
  line L1523 (-135.8501, 21.35) -> (-135.8501, 24.35)
  line L1524 (-135.8501, 24.35) -> (-138.8501, 24.35)
  line L1525 (-138.8501, 24.35) -> (-138.8501, 21.35)
  line L1526 (-138.8501, 21.35) -> (-141.8501, 21.35)
  line L1527 (-141.8501, 21.35) -> (-141.8501, 24.35)
  line L1528 (-141.8501, 24.35) -> (-144.8501, 24.35)
  line L1529 (-144.8501, 24.35) -> (-144.8501, 21.35)
  line L1530 (-144.8501, 21.35) -> (-147.8501, 21.35)
  line L1531 (-147.8501, 21.35) -> (-147.8501, 24.35)
  line L1532 (-147.8501, 24.35) -> (-150.8501, 24.35)
  line L1533 (-150.8501, 24.35) -> (-150.8501, 21.35)
  line L1534 (-150.8501, 21.35) -> (-153.8501, 21.35)
  line L1535 (-153.8501, 21.35) -> (-153.8501, 24.35)
  line L1536 (-153.8501, 24.35) -> (-156.8501, 24.35)
  line L1537 (-156.8501, 24.35) -> (-156.8501, 21.35)
  line L1538 (-156.8501, 21.35) -> (-159.8501, 21.35)
  line L1539 (-159.8501, 21.35) -> (-159.8501, 24.35)
  line L1540 (-159.8501, 24.35) -> (-162.8501, 24.35)
  line L1541 (-162.8501, 24.35) -> (-162.8501, 21.35)
  line L1542 (-162.8501, 21.35) -> (-165.8501, 21.35)
  line L1543 (-165.8501, 21.35) -> (-165.8501, 24.35)
  line L1544 (-165.8501, 24.35) -> (-168.8501, 24.35)
  line L1545 (-168.8501, 24.35) -> (-168.8501, 21.35)
  line L1546 (-168.8501, 21.35) -> (-171.8501, 21.35)
  line L1547 (-171.8501, 21.35) -> (-171.8501, 24.35)
  line L1548 (-171.8501, 24.35) -> (-174.8501, 24.35)
  line L1549 (-174.8501, 24.35) -> (-174.8501, 21.35)
  line L1550 (-174.8501, 21.35) -> (-177.8501, 21.35)
  line L1551 (-177.8501, 21.35) -> (-177.8501, 24.35)
  line L1552 (-177.8501, 24.35) -> (-180.8501, 24.35)
  line L1553 (-180.8501, 24.35) -> (-180.8501, 21.35)
  line L1554 (-180.8501, 21.35) -> (-183.8502, 21.35)
  line L1555 (-183.8502, 21.35) -> (-183.8502, 24.35)
  line L1556 (-183.8502, 24.35) -> (-186.8502, 24.35)
  line L1557 (-186.8502, 24.35) -> (-186.8502, 21.35)
  line L1558 (-186.8502, 21.35) -> (-189.8502, 21.35)
  line L1559 (-189.8502, 21.35) -> (-189.8502, 24.35)
  line L1560 (-189.8502, 24.35) -> (-192.8502, 24.35)
  line L1561 (-192.8502, 24.35) -> (-192.8502, 21.35)
  line L1562 (-192.8502, 21.35) -> (-195.8502, 21.35)
  line L1563 (-195.8502, 21.35) -> (-195.8502, 24.35)
  line L1564 (-195.8502, 24.35) -> (-198.8502, 24.35)
  line L1565 (-198.8502, 24.35) -> (-198.8502, 21.35)
  line L1566 (-198.8502, 21.35) -> (-201.8502, 21.35)
  line L1567 (-201.8502, 21.35) -> (-201.8502, 24.35)
  line L1568 (-201.8502, 24.35) -> (-204.8502, 24.35)
  line L1569 (-204.8502, 24.35) -> (-204.8502, 21.35)
  line L1570 (-204.8502, 21.35) -> (-207.8502, 21.35)
  line L1571 (-207.8502, 21.35) -> (-207.8502, 24.35)
  line L1572 (-207.8502, 24.35) -> (-210.8502, 24.35)
  line L1573 (-210.8502, 24.35) -> (-210.8502, 21.35)
  line L1574 (-210.8502, 21.35) -> (-213.8502, 21.35)
  line L1575 (-213.8502, 21.35) -> (-213.8502, 24.35)
  line L1576 (-213.8502, 24.35) -> (-216.8502, 24.35)
  line L1577 (-216.8502, 24.35) -> (-216.8502, 21.35)
  line L1578 (-216.8502, 21.35) -> (-219.8502, 21.35)
  line L1579 (-219.8502, 21.35) -> (-219.8502, 24.35)
  line L1580 (-219.8502, 24.35) -> (-222.8502, 24.35)
  line L1581 (-222.8502, 24.35) -> (-222.8502, 21.35)
  line L1582 (-222.8502, 21.35) -> (-225.8502, 21.35)
  line L1583 (-225.8502, 21.35) -> (-225.8502, 24.35)
  line L1584 (-225.8502, 24.35) -> (-228.8502, 24.35)
  line L1585 (-228.8502, 24.35) -> (-228.8502, 21.35)
  line L1586 (-228.8502, 21.35) -> (-231.8502, 21.35)
  line L1587 (-231.8502, 21.35) -> (-231.8502, 24.35)
  line L1588 (-231.8502, 24.35) -> (-234.8502, 24.35)
  line L1589 (-234.8502, 24.35) -> (-234.8502, 21.35)
  line L1590 (-234.8502, 21.35) -> (-237.8502, 21.35)
  line L1591 (-237.8502, 21.35) -> (-237.8502, 24.35)
  line L1592 (-237.8502, 24.35) -> (-240.8502, 24.35)
  line L1593 (-240.8502, 24.35) -> (-240.8502, 21.35)
  line L1594 (-240.8502, 21.35) -> (-243.8502, 21.35)
  line L1595 (-243.8502, 21.35) -> (-243.8502, 24.35)
  line L1596 (-243.8502, 24.35) -> (-246.8502, 24.35)
  line L1597 (-246.8502, 24.35) -> (-246.8502, 21.35)
  line L1598 (-246.8502, 21.35) -> (-249.8502, 21.35)
  line L1599 (-249.8502, 21.35) -> (-249.8502, 24.35)
  line L1600 (-249.8502, 24.35) -> (-252.8502, 24.35)
  line L1601 (-252.8502, 24.35) -> (-252.8502, 21.35)
  line L1602 (-252.8502, 21.35) -> (-255.8502, 21.35)
  line L1603 (-255.8502, 21.35) -> (-255.8502, 24.35)
  line L1604 (-255.8502, 24.35) -> (-258.8502, 24.35)
  line L1605 (-258.8502, 24.35) -> (-258.8502, 21.35)
  line L1606 (-258.8502, 21.35) -> (-261.8502, 21.35)
  line L1607 (-261.8502, 21.35) -> (-261.8502, 24.35)
  line L1608 (-261.8502, 24.35) -> (-264.8502, 24.35)
  line L1609 (-264.8502, 24.35) -> (-264.8502, 21.35)
  line L1610 (-264.8502, 21.35) -> (-267.8502, 21.35)
  line L1611 (-267.8502, 21.35) -> (-267.8502, 24.35)
  line L1612 (-267.8502, 24.35) -> (-270.8502, 24.35)
  line L1613 (-270.8502, 24.35) -> (-270.8502, 21.35)
  line L1614 (-270.8502, 21.35) -> (-273.8502, 21.35)
  line L1615 (-273.8502, 21.35) -> (-273.8502, 24.35)
  line L1616 (-273.8502, 24.35) -> (-276.8502, 24.35)
  line L1617 (-276.8502, 24.35) -> (-276.8502, 21.35)
  line L1618 (-276.8502, 21.35) -> (-279.8502, 21.35)
  line L1619 (-279.8502, 21.35) -> (-279.8502, 24.35)
  line L1620 (-279.8502, 24.35) -> (-282.8502, 24.35)
  line L1621 (-282.8502, 24.35) -> (-282.8502, 21.35)
  line L1622 (-282.8502, 21.35) -> (-285.8502, 21.35)
  line L1623 (-285.8502, 21.35) -> (-285.8502, 24.35)
  line L1624 (-285.8502, 24.35) -> (-288.8502, 24.35)
  line L1625 (-288.8502, 24.35) -> (-288.8502, 21.35)
  line L1626 (-288.8502, 21.35) -> (-291.8502, 21.35)
  line L1627 (-291.8502, 21.35) -> (-291.8502, 24.35)
  line L1628 (-291.8502, 24.35) -> (-294.8502, 24.35)
  line L1629 (-294.8502, 24.35) -> (-294.8502, 21.35)
  line L1630 (-294.8502, 21.35) -> (-297.8502, 21.35)
  line L1631 (-297.8502, 21.35) -> (-297.8502, 24.35)
  line L1632 (-297.8502, 24.35) -> (-300.8502, 24.35)
  line L1633 (-300.8502, 24.35) -> (-300.8502, 21.35)
  line L1634 (-300.8502, 21.35) -> (-303.8502, 21.35)
  line L1635 (-303.8502, 21.35) -> (-303.8502, 24.35)
  line L1636 (-303.8502, 24.35) -> (-306.8503, 24.35)
  line L1637 (-306.8503, 24.35) -> (-306.8503, 21.35)
  line L1638 (-306.8503, 21.35) -> (-309.8503, 21.35)
  line L1639 (-309.8503, 21.35) -> (-309.8503, 24.35)
  line L1640 (-309.8503, 24.35) -> (-312.8503, 24.35)
  line L1641 (-312.8503, 24.35) -> (-312.8503, 21.35)
  line L1642 (-312.8503, 21.35) -> (-317.6003, 21.35)
  line L1643 (-317.6003, 21.35) -> (-317.6003, 24.35)
  line L1644 (-317.6003, 24.35) -> (-322.3503, 24.35)
  line L1645 (-322.3503, 24.35) -> (-322.3503, 20.6)
  line L1646 (-322.3503, 20.6) -> (-319.3503, 20.6)
  line L1647 (-319.3503, 20.6) -> (-319.3503, 16.85)
  line L1648 (-319.3503, 16.85) -> (-322.3503, 16.85)
  line L1649 (-322.3503, 16.85) -> (-322.3503, 13.85)
  line L1650 (-322.3503, 13.85) -> (-319.3503, 13.85)
  line L1651 (-319.3503, 13.85) -> (-319.3503, 10.1)
  line L1652 (-620.3505, 37.3501) -> (-620.3505, 167.3501)
  line L1653 (-620.3505, 167.3501) -> (-390.3505, 167.3501)
  line L1654 (-390.3505, 167.3501) -> (-390.3505, 37.3501)
  line L1655 (-390.3505, 37.3501) -> (-620.3505, 37.3501)
  line L1656 (-325.3503, 28.1) -> (-322.3503, 28.1)
  line L1657 (-322.3503, 28.1) -> (-322.3503, 31.85)
  line L1658 (-322.3503, 31.85) -> (-325.3503, 31.85)
  line L1659 (-325.3503, 31.85) -> (-325.3503, 34.85)
  line L1660 (-325.3503, 34.85) -> (-322.3503, 34.85)
  line L1661 (-322.3503, 34.85) -> (-322.3503, 37.85)
  line L1662 (-322.3503, 37.85) -> (-325.3503, 37.85)
  line L1663 (-325.3503, 37.85) -> (-325.3503, 40.85)
  line L1664 (-325.3503, 40.85) -> (-322.3503, 40.85)
  line L1665 (-322.3503, 40.85) -> (-322.3503, 43.85)
  line L1666 (-322.3503, 43.85) -> (-325.3503, 43.85)
  line L1667 (-325.3503, 43.85) -> (-325.3503, 46.85)
  line L1668 (-325.3503, 46.85) -> (-322.3503, 46.85)
  line L1669 (-322.3503, 46.85) -> (-322.3503, 49.85)
  line L1670 (-322.3503, 49.85) -> (-325.3503, 49.85)
  line L1671 (-325.3503, 49.85) -> (-325.3503, 52.85)
  line L1672 (-325.3503, 52.85) -> (-322.3503, 52.85)
  line L1673 (-322.3503, 52.85) -> (-322.3503, 55.85)
  line L1674 (-322.3503, 55.85) -> (-325.3503, 55.85)
  line L1675 (-325.3503, 55.85) -> (-325.3503, 58.85)
  line L1676 (-325.3503, 58.85) -> (-322.3503, 58.85)
  line L1677 (-322.3503, 58.85) -> (-322.3503, 61.8501)
  line L1678 (-322.3503, 61.8501) -> (-325.3503, 61.8501)
  line L1679 (-325.3503, 61.8501) -> (-325.3503, 64.8501)
  line L1680 (-325.3503, 64.8501) -> (-322.3503, 64.8501)
  line L1681 (-322.3503, 64.8501) -> (-322.3503, 67.8501)
  line L1682 (-322.3503, 67.8501) -> (-325.3503, 67.8501)
  line L1683 (-325.3503, 67.8501) -> (-325.3503, 70.8501)
  line L1684 (-325.3503, 70.8501) -> (-322.3503, 70.8501)
  line L1685 (-322.3503, 70.8501) -> (-322.3503, 73.8501)
  line L1686 (-322.3503, 73.8501) -> (-325.3503, 73.8501)
  line L1687 (-325.3503, 73.8501) -> (-325.3503, 76.8501)
  line L1688 (-325.3503, 76.8501) -> (-322.3503, 76.8501)
  line L1689 (-322.3503, 76.8501) -> (-322.3503, 79.8501)
  line L1690 (-322.3503, 79.8501) -> (-325.3503, 79.8501)
  line L1691 (-325.3503, 79.8501) -> (-325.3503, 82.8501)
  line L1692 (-325.3503, 82.8501) -> (-322.3503, 82.8501)
  line L1693 (-322.3503, 82.8501) -> (-322.3503, 85.8501)
  line L1694 (-322.3503, 85.8501) -> (-325.3503, 85.8501)
  line L1695 (-325.3503, 85.8501) -> (-325.3503, 88.8501)
  line L1696 (-325.3503, 88.8501) -> (-322.3503, 88.8501)
  line L1697 (-322.3503, 88.8501) -> (-322.3503, 91.8501)
  line L1698 (-322.3503, 91.8501) -> (-325.3503, 91.8501)
  line L1699 (-325.3503, 91.8501) -> (-325.3503, 94.8501)
  line L1700 (-325.3503, 94.8501) -> (-322.3503, 94.8501)
  line L1701 (-322.3503, 94.8501) -> (-322.3503, 97.8501)
  line L1702 (-322.3503, 97.8501) -> (-325.3503, 97.8501)
  line L1703 (-325.3503, 97.8501) -> (-325.3503, 100.8501)
  line L1704 (-325.3503, 100.8501) -> (-322.3503, 100.8501)
  line L1705 (-322.3503, 100.8501) -> (-322.3503, 103.8501)
  line L1706 (-322.3503, 103.8501) -> (-325.3503, 103.8501)
  line L1707 (-325.3503, 103.8501) -> (-325.3503, 106.8501)
  line L1708 (-325.3503, 106.8501) -> (-322.3503, 106.8501)
  line L1709 (-322.3503, 106.8501) -> (-322.3503, 109.8501)
  line L1710 (-322.3503, 109.8501) -> (-325.3503, 109.8501)
  line L1711 (-325.3503, 109.8501) -> (-325.3503, 112.8501)
  line L1712 (-325.3503, 112.8501) -> (-322.3503, 112.8501)
  line L1713 (-322.3503, 112.8501) -> (-322.3503, 115.8501)
  line L1714 (-322.3503, 115.8501) -> (-325.3503, 115.8501)
  line L1715 (-325.3503, 115.8501) -> (-325.3503, 118.8501)
  line L1716 (-325.3503, 118.8501) -> (-322.3503, 118.8501)
  line L1717 (-322.3503, 118.8501) -> (-322.3503, 121.8501)
  line L1718 (-322.3503, 121.8501) -> (-325.3503, 121.8501)
  line L1719 (-325.3503, 121.8501) -> (-325.3503, 124.8501)
  line L1720 (-325.3503, 124.8501) -> (-322.3503, 124.8501)
  line L1721 (-322.3503, 124.8501) -> (-322.3503, 127.8501)
  line L1722 (-322.3503, 127.8501) -> (-325.3503, 127.8501)
  line L1723 (-325.3503, 127.8501) -> (-325.3503, 130.8501)
  line L1724 (-325.3503, 130.8501) -> (-322.3503, 130.8501)
  line L1725 (-322.3503, 130.8501) -> (-322.3503, 133.8501)
  line L1726 (-322.3503, 133.8501) -> (-325.3503, 133.8501)
  line L1727 (-325.3503, 133.8501) -> (-325.3503, 136.8501)
  line L1728 (-325.3503, 136.8501) -> (-322.3503, 136.8501)
  line L1729 (-322.3503, 136.8501) -> (-322.3503, 139.8501)
  line L1730 (-322.3503, 139.8501) -> (-325.3503, 139.8501)
  line L1731 (-325.3503, 139.8501) -> (-325.3503, 142.8501)
  line L1732 (-325.3503, 142.8501) -> (-322.3503, 142.8501)
  line L1733 (-322.3503, 142.8501) -> (-322.3503, 145.8501)
  line L1734 (-322.3503, 145.8501) -> (-325.3503, 145.8501)
  line L1735 (-325.3503, 145.8501) -> (-325.3503, 148.8501)